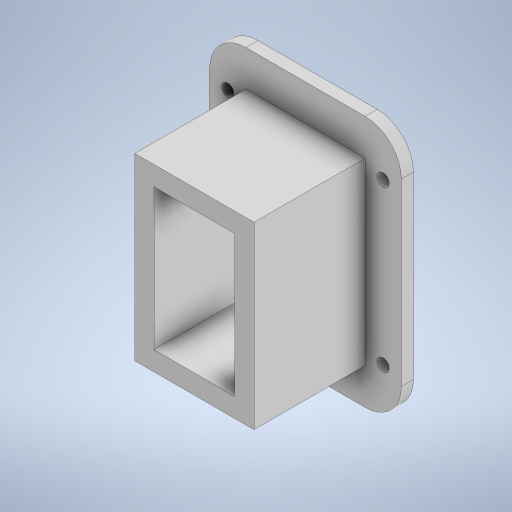
# Autodesk Inventor part: Base_Demo_1
Saved by Autodesk Inventor 2023.5 (Build 275446020, 446B)
## iProperties
Created: 2025-04-11
Part Number: Base_Demo_1
Material: Generic
Document SubType Name: Modeling
Designer: Lucky
Density: 1 g/cm^3
Appearance: Default
Author: Lucky
Autodesk Inventor part; units mm, degrees
ref_plane "YZ Plane" through (0, 0, 0) normal (1, 0, 0) x (0, 1, 0)
ref_plane "XZ Plane" through (0, 0, 0) normal (0, 1, 0) x (-1, 0, 0)
ref_plane "XY Plane" through (0, 0, 0) normal (0, 0, 1) x (1, 0, 0)
sketch "Sketch1" plane through (0, 0, 0) normal (0, 0, 1) x (1, 0, 0)
  line L0 (0, 0) -> (33.4, 0)
  line L1 (33.4, 0) -> (33.4, 58.4)
  line L2 (33.4, 58.4) -> (0, 58.4)
  line L3 (0, 58.4) -> (0, 0)
  line L4 (-8, 66.4) -> (41.4, 66.4)
  line L5 (41.4, 66.4) -> (41.4, -8)
  line L6 (41.4, -8) -> (-8, -8)
  line L7 (-8, -8) -> (-8, 66.4)
  line L8 (56.4, -8) -> (56.4, 66.4)
  line L9 (41.4, 81.4) -> (-8, 81.4)
  line L10 (-23, 66.4) -> (-23, -8)
  line L11 (-8, -23) -> (41.4, -23)
  circle A0 centre (48.9, 62.4) radius 2.55
  circle A1 centre (48.9, -4) radius 2.55
  circle A2 centre (-15.5, 62.4) radius 2.55
  circle A3 centre (-15.5, -4) radius 2.55
  arc A4 (-8, 81.4) -> (-23, 66.4) centre (-8, 66.4) ccw
  arc A5 (56.4, 66.4) -> (41.4, 81.4) centre (41.4, 66.4) ccw
  arc A6 (41.4, -23) -> (56.4, -8) centre (41.4, -8) ccw
  arc A7 (-23, -8) -> (-8, -23) centre (-8, -8) ccw
  dimension "d0" = 58.4
  dimension "d1" = 33.4
  dimension "d2" = 8
  dimension "d3" = 15
  dimension "d4" = 5.1
  dimension "d5" = 7.5
  dimension "d6" = 5.1
  dimension "d7" = 5.1
  dimension "d8" = 7.5
  dimension "d9" = 5.1
  dimension "d10" = 4
  dimension "d11" = 4
  dimension "d12" = 4
  dimension "d13" = 4
  dimension "d14" = 7.5
  dimension "d15" = 7.5
  dimension "d16" = 15
  constraints: 24 end point, 8 centre point, 8 point on circle, 8 tangent, 6 parallel, 3 equal radius, 3 perpendicular, 1 horizontal, 6 other
  measures "d0" distance between parallel lines of L0 L2
  measures "d1" distance between parallel lines of L1 L3
  measures "d2" distance between parallel lines of L2 L4
  measures "d3" distance between parallel lines of L5 L8
  measures "d4" diameter of A0
  measures "d5" distance from line of L5 A0.centre
  measures "d6" diameter of A1
  measures "d7" diameter of A2
  measures "d8" distance from line of L7 A2.centre
  measures "d9" diameter of A3
  measures "d10" distance from line of L4 A0.centre
  measures "d11" distance from line of L6 A1.centre
  measures "d12" distance from line of L4 A2.centre
  measures "d13" distance from line of L6 A3.centre
  measures "d14" distance from line of L7 A3.centre
  measures "d15" distance from line of L8 A1.centre
  measures "d16" radius of A4
extrude "Extrusion1" add sketch "Sketch1" against normal blind 46 contours L4 L5 L6 L7
sketch "Sketch2" plane through (0, 0, -46) normal (0, 0, -1) x (-1, 0, 0)
  line L0 (-41.4, 66.4) -> (8, 66.4)
  line L1 (8, 66.4) -> (8, -8)
  line L2 (8, -8) -> (-41.4, -8)
  line L3 (-41.4, -8) -> (-41.4, 66.4)
  line L4 (8, 81.4) -> (-41.4, 81.4)
  line L5 (-56.4, 66.4) -> (-56.4, -8)
  line L6 (-41.4, -23) -> (8, -23)
  line L7 (23, -8) -> (23, 66.4)
  circle A0 centre (-48.9, 62.4) radius 2.55
  circle A1 centre (15.5, 62.4) radius 2.55
  circle A2 centre (-48.9, -4) radius 2.55
  circle A3 centre (15.5, -4) radius 2.55
  arc A4 (-56.4, -8) -> (-41.4, -23) centre (-41.4, -8) ccw
  arc A5 (23, 66.4) -> (8, 81.4) centre (8, 66.4) ccw
  arc A6 (-41.4, 81.4) -> (-56.4, 66.4) centre (-41.4, 66.4) ccw
  arc A7 (8, -23) -> (23, -8) centre (8, -8) ccw
  point P0 (0, 0)
  dimension "d19" = 15
  dimension "d20" = 5.1
  dimension "d21" = 5.1
  dimension "d22" = 4
  dimension "d23" = 4
  dimension "d24" = 7.5
  dimension "d25" = 7.5
  dimension "d26" = 5.1
  dimension "d27" = 4
  dimension "d28" = 7.5
  dimension "d29" = 5.1
  dimension "d30" = 4
  dimension "d31" = 7.5
  dimension "d32" = 15
  constraints: 16 end point, 8 centre point, 8 point on circle, 8 tangent, 4 parallel, 3 equal radius, 2 perpendicular, 1 horizontal, 3 other
  measures "d19" distance between parallel lines of L0 L4
  measures "d20" diameter of A0
  measures "d21" diameter of A1
  measures "d22" distance from line of L0 A1.centre
  measures "d23" distance from line of L0 A0.centre
  measures "d24" distance from line of L1 A1.centre
  measures "d25" distance from line of L5 A0.centre
  measures "d26" diameter of A2
  measures "d27" distance from line of L2 A2.centre
  measures "d28" distance from line of L3 A2.centre
  measures "d29" diameter of A3
  measures "d30" distance from line of L2 A3.centre
  measures "d31" distance from line of L1 A3.centre
  measures "d32" radius of A4
extrude "Extrusion2" add sketch "Sketch2" along normal blind 5 contours L0 L1 L2 L3 | A5 L7 A7 L6 A4 L5 A6 L4
body "Solid1"
